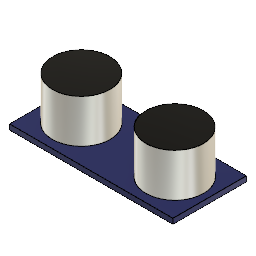
Ultrasonic v3 (Autodesk Fusion 360 design; units mm, degrees)
Autodesk Fusion 360 part; units mm, degrees
box "BoxPrimitive1" add length 20.5 width 45.5 height 1.5 placed x (0, 1, 0) y (-1, 0, 0) z (0, 0, 1) at (45.5, 0, 0)
sketch "Sketch2" plane through (0, 0, 1.5) normal (0, 0, 1) x (-1, 0, 0)
  line L0 (-45.5, -20.5) -> (0, -20.5)
  line L1 (0, -20.5) -> (0, 0)
  line L2 (0, 0) -> (-45.5, 0)
  line L3 (-45.5, 0) -> (-45.5, -20.5)
  line L4 (-45.5, -20.5) -> (-35.75, -20.5)
  line L5 (-35.75, -20.5) -> (-35.75, -10.25)
  line L6 (0, -20.5) -> (-9.75, -20.5)
  line L7 (-9.75, -20.5) -> (-9.75, -10.25)
  dimension "d6" = 9.75
  dimension "d7" = 10.25
  dimension "d10" = 9.75
  dimension "d11" = 10.25
  constraint coincident L0.start L3.end
  constraint perpendicular L3 L4
  constraint perpendicular L4 L5
  constraint coincident L0.end L1.start
  constraint coincident L0 L6.end
  constraint perpendicular L6 L7
  measures "d6" distance of L0.start L4.end
  measures "d7" distance of L4.end L5.end
  measures "d10" distance of L0.end L6.end
  measures "d11" distance of L6.end L7.end
cylinder "CylinderPrimitive1" add diameter 16 height 12 placed x (1, 0, 0) y (0, 1, 0) z (0, 0, 1) at (35.75, 10.25, 1.5)
cylinder "CylinderPrimitive2" add diameter 16 height 12 placed x (1, 0, 0) y (0, 1, 0) z (0, 0, 1) at (9.75, 10.25, 1.5)
